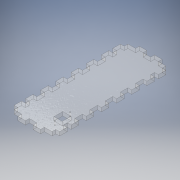
# Autodesk Inventor part: case_front
Saved by Autodesk Inventor 2019 (Build 230136000, 136)
## iProperties
Created: 2019-02-02
Part Number: case_front
Material: Acrylic, Clear
Document SubType Name: Modeling
Designer: suchanek
Density: 1.19 g/cm^3
Appearance: Transparent - Clear
Author: suchanek
Autodesk Inventor part; units mm, degrees
ref_plane "YZ Plane" through (0, 0, 0) normal (1, 0, 0) x (0, 1, 0)
ref_plane "XZ Plane" through (0, 0, 0) normal (0, 1, 0) x (-1, 0, 0)
ref_plane "XY Plane" through (0, 0, 0) normal (0, 0, 1) x (1, 0, 0)
sketch "Sketch1" plane through (0, 0, 0) normal (0, 1, 0) x (-1, 0, 0)
  line L0 (-30, 90) -> (30, 90)
  line L1 (30, 90) -> (30, -90)
  line L2 (30, -90) -> (-30, -90)
  line L3 (-30, -90) -> (-30, 90)
  line L4 (-30, 90) -> (30, -90) construction
  line L5 (30, 90) -> (-30, -90) construction
  line L6 (-30, 84) -> (-36, 84)
  line L7 (-36, 84) -> (-36, 72)
  line L8 (-36, 72) -> (-30, 72)
  line L9 (-30, 72) -> (-30, 84)
  line L10 (-36, 66) -> (-30, 66)
  line L11 (-30, 66) -> (-30, 54)
  line L12 (-30, 54) -> (-36, 54)
  line L13 (-36, 54) -> (-36, 66)
  line L14 (-30, 42) -> (-36, 42)
  line L15 (-36, 42) -> (-36, 30)
  line L16 (-36, 30) -> (-30, 30)
  line L17 (-30, 30) -> (-30, 42)
  line L18 (-30, 18) -> (-36, 18)
  line L19 (-36, 18) -> (-36, 6)
  line L20 (-36, 6) -> (-30, 6)
  line L21 (-30, 6) -> (-30, 18)
  line L22 (0, 0) -> (-5.6352, 0)
  line L23 (-5.6352, 0) -> (0, 0)
  line L24 (0, 0) -> (0, 8.7024)
  line L25 (-30, 90) -> (30, -90) construction
  line L26 (30, 84) -> (36, 84)
  line L27 (36, 84) -> (36, 72)
  line L28 (36, 72) -> (30, 72)
  line L29 (30, 72) -> (30, 84)
  line L30 (36, 66) -> (30, 66)
  line L31 (30, 66) -> (30, 54)
  line L32 (30, 54) -> (36, 54)
  line L33 (36, 54) -> (36, 66)
  line L34 (30, 42) -> (36, 42)
  line L35 (36, 42) -> (36, 30)
  line L36 (36, 30) -> (30, 30)
  line L37 (30, 30) -> (30, 42)
  line L38 (30, 18) -> (36, 18)
  line L39 (36, 18) -> (36, 6)
  line L40 (36, 6) -> (30, 6)
  line L41 (30, 6) -> (30, 18)
  line L42 (-30, -84) -> (-36, -84)
  line L43 (-36, -84) -> (-36, -72)
  line L44 (-36, -72) -> (-30, -72)
  line L45 (-30, -72) -> (-30, -84)
  line L46 (-36, -66) -> (-30, -66)
  line L47 (-30, -66) -> (-30, -54)
  line L48 (-30, -54) -> (-36, -54)
  line L49 (-36, -54) -> (-36, -66)
  line L50 (-30, -42) -> (-36, -42)
  line L51 (-36, -42) -> (-36, -30)
  line L52 (-36, -30) -> (-30, -30)
  line L53 (-30, -30) -> (-30, -42)
  line L54 (-30, -18) -> (-36, -18)
  line L55 (-36, -18) -> (-36, -6)
  line L56 (-36, -6) -> (-30, -6)
  line L57 (-30, -6) -> (-30, -18)
  line L58 (36, -42) -> (36, -30)
  line L59 (30, -30) -> (30, -42)
  line L60 (30, -6) -> (30, -18)
  line L61 (36, -6) -> (30, -6)
  line L62 (36, -18) -> (36, -6)
  line L63 (30, -18) -> (36, -18)
  line L64 (36, -30) -> (30, -30)
  line L65 (30, -84) -> (36, -84)
  line L66 (36, -84) -> (36, -72)
  line L67 (36, -72) -> (30, -72)
  line L68 (30, -72) -> (30, -84)
  line L69 (30, -42) -> (36, -42)
  line L70 (30, -54) -> (36, -54)
  line L71 (30, -66) -> (30, -54)
  line L72 (36, -66) -> (30, -66)
  line L73 (36, -54) -> (36, -66)
  line L74 (18, 90) -> (6, 90)
  line L75 (6, 90) -> (6, 96)
  line L76 (6, 96) -> (18, 96)
  line L77 (18, 96) -> (18, 90)
  line L78 (-18, 90) -> (-6, 90)
  line L79 (-6, 90) -> (-6, 96)
  line L80 (-6, 96) -> (-18, 96)
  line L81 (-18, 96) -> (-18, 90)
  line L82 (18, -90) -> (6, -90)
  line L83 (6, -90) -> (6, -96)
  line L84 (6, -96) -> (18, -96)
  line L85 (18, -96) -> (18, -90)
  line L86 (-18, -90) -> (-6, -90)
  line L87 (-6, -90) -> (-6, -96)
  line L88 (-6, -96) -> (-18, -96)
  line L89 (-18, -96) -> (-18, -90)
  line L90 (-11, 68) -> (-24, 68)
  line L91 (-24, 68) -> (-24, 54)
  line L92 (-24, 54) -> (-11, 54)
  line L93 (-11, 54) -> (-11, 68)
  circle A0 centre (-17.5, 49) radius 1
  circle A1 centre (-17.5, 73) radius 1
  line L94 (-17.5, 73) -> (-17.5, 49)
  point P0 (0, -8.7024)
  dimension "d0" = 60
  dimension "d1" = 180
  dimension "d2" = 6
  dimension "d3" = 6
  dimension "d4" = 12
  dimension "d5" = 12
  dimension "d6" = 12
  dimension "d7" = 12
  dimension "d8" = 12
  dimension "d9" = 6
  dimension "d10" = 12
  dimension "d17" = 6
  dimension "d19" = 6
  dimension "d20" = 12
  dimension "d24" = 6
  dimension "d25" = 13
  dimension "d26" = 14
  dimension "d27" = 22
  dimension "d28" = 2
  dimension "d30" = 5
  dimension "d31" = 5
  constraints: 190 end point, 61 symmetric about line, 17 point on line, 15 equal length, 8 horizontal, 7 perpendicular, 2 centre point, 2 midpoint, 2 vertical, 1 equal radius, 1 other
  measures "d0" distance of L1.end L2.end
  measures "d1" distance of L0.end L1.end
  measures "d2" distance of L19.end L20.end
  measures "d3" distance from line of L22.start L20
  measures "d4" distance of L18.end L19.end
  measures "d5" distance between parallel lines of L18 L16
  measures "d6" distance of L14.end L15.end
  measures "d7" distance between parallel lines of L12 L14
  measures "d8" distance of L12.end L10.start
  measures "d9" distance between parallel lines of L10 L8
  measures "d10" distance of L6.end L7.end
  measures "d17" distance of L74.end L75.end
  measures "d19" distance between parallel lines of L24 L75
  measures "d20" distance of L75.end L76.end
  measures "d24" distance between parallel lines of L3 L91
  measures "d25" distance of L90.start L90.end
  measures "d26" distance of L92.end L90.start
  measures "d27" distance from line of L78.start L90
  measures "d28" diameter of A0
  measures "d30" distance from line of L92 L94.end
  measures "d31" distance from line of L90 L94.start
extrude "Extrusion1" add sketch "Sketch1" along normal blind 6
body "Solid1"
